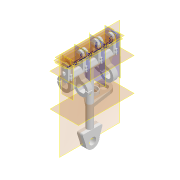
# Autodesk Inventor part: base_hand
Saved by Autodesk Inventor 2020.2 (Build 242310000, 310)
## iProperties
Created: 2020-04-08
Part Number: base_hand
Material: Generic
Document SubType Name: Modeling
Designer: Bardo91
Density: 1 g/cm^3
Appearance: Default
Author: Bardo91
Autodesk Inventor part; units mm, degrees
sketch "Sketch1" plane through (0, 0, 0) normal (1, 0, 0) x (0, 1, 0)
  line L0 (0, 0) -> (0, -22)
  line L1 (0, -22) -> (0, -44)
  line L2 (0, -44) -> (0, -66)
  line L3 (0, -22) -> (5, -22)
  line L4 (0, -44) -> (8, -44)
  line L5 (0, -66) -> (5, -66)
  dimension "d0" = 22
  dimension "d1" = 22
  dimension "d2" = 22
  dimension "d4" = 5
  dimension "d5" = 8
  dimension "d6" = 5
  constraints: 12 end point, 2 horizontal, 2 point on line, 1 perpendicular, 1 vertical
  measures "d0" distance of L0.start L0.end
  measures "d1" distance of L0.end L1.end
  measures "d2" distance of L1.end L2.end
  measures "d4" distance of L0.end L3.end
  measures "d5" distance of L1.end L4.end
  measures "d6" distance of L2.end L5.end
ref_plane "Work Plane1" through (0, 5, -22) normal (0, 0, 1) x (1, 0, 0)
ref_plane "Work Plane3" through (0, 5, -66) normal (0, 0, 1) x (1, 0, 0)
ref_plane "Work Plane2" through (0, 8, -44) normal (0, 0, 1) x (1, 0, 0)
ref_plane "Work Plane4" through (0, 0, 0) normal (0, 0, 1) x (1, 0, 0)
sketch "Sketch2" plane through (0, 0, 0) normal (0, 0, 1) x (1, 0, 0)
  circle A0 centre (0, 0) radius 1.5
  circle A1 centre (0, 0) radius 5
  line L0 (0, 0) -> (0, -15)
  circle A2 centre (0, -15) radius 5
  line L1 (5, -15) -> (5, 0)
  line L2 (-5, -15) -> (-5, 0)
  dimension "d7" = 3
  dimension "d8" = 10
  dimension "d80" = 15
  dimension "d81" = 10
  constraints: 6 end point, 4 point on circle, 3 centre point, 3 coincident, 2 tangent, 2 vertical, 1 parallel
  measures "d7" diameter of A0
  measures "d8" diameter of A1
  measures "d80" distance of L0.start L0.end
  measures "d81" diameter of A2
extrude "pinky_joint" add sketch "Sketch2" along normal mid plane 8
sketch "Sketch18" plane through (0, 0, 4) normal (0, 0, 1) x (1, 0, 0)
  line L0 (0, 0) -> (0, -6)
  line L1 (0, -6) -> (0, -9)
  line L2 (0, 0) -> (1.058, -6)
  line L3 (0, 0) -> (6.0926, 0) construction
  line L4 (1.058, -6) -> (0, -6)
  line L5 (1.058, -6) -> (1.5869, -9)
  line L6 (1.5869, -9) -> (0, -9)
  dimension "d82" = 6
  dimension "d83" = 3
  dimension "d84" = 80
  constraints: 14 end point, 2 horizontal, 2 point on line, 1 equal length, 1 parallel, 1 vertical
  measures "d82" distance of L0.start L0.end
  measures "d83" distance of L0.end L1.end
  measures "d84" angle of L2 L3
extrude "lock" add sketch "Sketch18" along normal blind 3 contours L4 L5 L6 L1
ref_plane "Work Plane5" through (0, 0, 0) normal (0, 0, 1) x (1, 0, 0)
mirror "Mirror1" about plane through (0, 0, 0) normal (0, 0, 1) of "lock"
chamfer "Chamfer1" distance 3 angle 45 2 edges at (0, -7.5, 4) (0, -7.5, -4)
ref_plane "Work Plane6" through (0, 5, 0) normal (0, 1, 0) x (-1, 0, 0)
sketch "Sketch19" plane through (0, 5, 0) normal (0, 1, 0) x (-1, 0, 0)
  line L0 (0, 0) -> (-3, 0)
  circle A0 centre (-3, 0) radius 1.25
  dimension "d90" = 3
  dimension "thread_hole" = 2.5
  constraints: 2 end point, 1 centre point, 1 coincident, 1 horizontal
  measures "d90" distance of L0.start L0.end
  measures "thread_hole" diameter of A0
extrude "thread_hole" cut sketch "Sketch19" against normal through all
sketch "Sketch20" plane through (0, 0, 0) normal (0, 1, 0) x (-1, 0, 0)
  line L0 (0, 0) -> (-3, 0)
  circle A0 centre (-3, 0) radius 1.25
  line L1 (-3, -1.25) -> (-5, -1.25)
  line L2 (-5, -4) -> (-5, 4) projected
  line L3 (-3, 1.25) -> (-5, 1.25)
  line L4 (0, 0) -> (0, 2.405)
  dimension "d94" = 3
  dimension "d95" = 2.5
  constraints: 8 end point, 2 horizontal, 2 point on circle, 2 point on line, 1 centre point, 1 coincident, 1 parallel, 1 vertical
  measures "d94" distance of L0.start L0.end
  measures "d95" diameter of A0
revolve "Revolution2" cut sketch "Sketch20" angle 180 about axis through (0, 0, 0) along (0, 0, 1)
sketch "Sketch22" plane through (5, -15, 4) normal (1, 0, 0) x (0, 0, -1)
  line L0 (8, 0) -> (0, 0) projected
  line L1 (4, 0) -> (4, 1)
  circle A0 centre (4, 1) radius 1
  line L2 (4, 1) -> (4, 5)
  circle A1 centre (4, 5) radius 1
  point P0 (4, 15)
  dimension "d100" = 1
  dimension "d101" = 2
  dimension "d104" = 4
  dimension "d105" = 2
  constraints: 4 end point, 2 centre point, 2 coincident, 2 vertical, 1 midpoint
  measures "d100" distance of L1.start L1.end
  measures "d101" diameter of A0
  measures "d104" distance of L2.start L2.end
  measures "d105" diameter of A1
extrude "pinky_flector_holder" cut sketch "Sketch22" against normal up to surface round surface about axis through (3, 5, 0) along (0, -1, 0) radius 1.25 far side no
sketch "Sketch23" plane through (0, 0, -4) normal (0, 0, -1) x (-1, 0, 0)
  arc A0 (-5, -15) -> (5, -15) centre (0, -15) ccw projected
  circle A1 centre (0, -15) radius 5
  point P0 (0, 0)
  constraints: 1 coincident, 3 other
extrude "finger_union" add sketch "Sketch23" along normal blind 66
sketch "Sketch24" plane through (-5, 0, -1.25) normal (0, 1, 0) x (1, 0, 0)
  arc A0 (2, -2.5) -> (2, 0) centre (2, -1.25) ccw projected
  circle A1 centre (2, -1.25) radius 1.25
  point P0 (5, -1.25)
  constraints: 1 coincident, 3 other
extrude "pinky_actuator_hole" cut sketch "Sketch24" against normal through all
ref_plane "Work Plane7" through (0, 5, -22) normal (0, 0, -1) x (-1, 0, 0)
sketch "Sketch25" plane through (0, 5, -22) normal (0, 0, -1) x (-1, 0, 0)
  arc A0 (5, -5) -> (-5, -5) centre (0, -5) ccw projected
  circle A1 centre (0, 0) radius 1.5
  circle A2 centre (0, 0) radius 5
  line L0 (5, -5) -> (5, -20) projected
  line L1 (5, 0) -> (5, -20)
  line L2 (-5, -20) -> (-5, -5) projected
  line L3 (-5, 0) -> (-5, -20)
  circle A3 centre (0, -20) radius 5 projected
  circle A4 centre (0, -20) radius 5
  point P0 (-5, -5)
  point P1 (5, -5)
  dimension "d112" = 3
  dimension "d113" = 10
  constraints: 4 end point, 3 point on circle, 2 centre point, 2 coincident, 2 collinear, 1 horizontal alignment, 2 other
  measures "d112" diameter of A1
  measures "d113" diameter of A2
extrude "ring_base" add sketch "Sketch25" along normal mid plane 8 contours L0 A3 L2 A0 A2 | A0 A2 L1 | A2 A0 A1 | A0 A1 A2 | A0 L3 A2
sketch "Sketch26" plane through (0, 5, -18) normal (0, 0, 1) x (1, 0, 0)
  line L0 (0, 0) -> (0, -6)
  line L1 (0, -6) -> (0, -9)
  line L2 (0, 0) -> (1.5869, -9)
  line L3 (0, 0) -> (9.1388, 0) construction
  line L4 (1.5869, -9) -> (0, -9)
  line L5 (0, -6) -> (1.058, -6)
  point P0 (0, -5)
  dimension "d116" = 6
  dimension "d117" = 3
  dimension "d118" = 80
  constraints: 12 end point, 2 horizontal, 2 vertical, 1 equal length, 1 parallel, 1 point on line
  measures "d116" distance of L0.start L0.end
  measures "d117" distance of L0.end L1.end
  measures "d118" angle of L2 L3
extrude "ring_lock" add sketch "Sketch26" along normal blind 3 contours L5 L2 L4 L1
mirror "Mirror2" about plane through (0, 5, -22) normal (0, 0, -1) of "ring_lock"
chamfer "Chamfer2" distance 3 angle 45 2 edges at (0, -2.5, -18) (0, -2.5, -26)
ref_plane "Work Plane8" through (0, 8, -44) normal (0, 0, -1) x (-1, 0, 0)
ref_plane "Work Plane9" through (0, 5, -66) normal (0, 0, -1) x (-1, 0, 0)
sketch "Sketch27" plane through (0, 8, -44) normal (0, 0, -1) x (-1, 0, 0)
  circle A0 centre (0, 0) radius 1.5
  circle A1 centre (0, 0) radius 5
  line L0 (5, -8) -> (5, -23) projected
  line L1 (5, 0) -> (5, -23)
  arc A2 (5, -23) -> (-5, -23) centre (0, -23) ccw projected
  line L2 (-5, 0) -> (-5, -23)
  point P0 (0, -8)
  point P1 (5, -8)
  dimension "d124" = 3
  dimension "d125" = 10
  constraints: 4 end point, 2 centre point, 2 point on circle, 2 vertical, 1 coincident, 1 tangent
  measures "d124" diameter of A0
  measures "d125" diameter of A1
extrude "middle_base" add sketch "Sketch27" along normal mid plane 8
ref_plane "Work Plane11" through (5, 8, -40) normal (0, 1, 0) x (-1, 0, 0)
ref_plane "Work Plane10" through (5, 5, -18) normal (0, 1, 0) x (-1, 0, 0)
sketch "Sketch28" plane through (0, 5, -66) normal (0, 0, -1) x (-1, 0, 0)
  circle A0 centre (0, 0) radius 1.5
  circle A1 centre (0, 0) radius 5
  line L0 (5, 3) -> (5, -20) projected
  line L1 (5, 0) -> (5, -20)
  line L2 (-5, -20) -> (-5, 3) projected
  line L3 (-5, 0) -> (-5, -20)
  arc A2 (5, -20) -> (-5, -20) centre (0, -20) ccw projected
  circle A3 centre (0, -20) radius 5
  point P0 (0, -5)
  dimension "d128" = 3
  dimension "d129" = 10
  constraints: 4 end point, 2 centre point, 2 coincident, 2 collinear, 2 point on circle, 2 point on line, 1 horizontal alignment, 1 tangent, 2 other
  measures "d128" diameter of A0
  measures "d129" diameter of A1
extrude "index_base" add sketch "Sketch28" along normal mid plane 8 contours A1 | L0 A2 L2 A1
sketch "Sketch39" plane through (5, 5, -18) normal (0, 1, 0) x (-1, 0, 0)
  line L0 (10, -8) -> (10, 0) projected
  line L1 (10, -4) -> (0, -4)
  line L2 (0, -8) -> (0, 0) projected
  line L3 (5, -4) -> (1.5, -4)
  circle A0 centre (1.5, -4) radius 1.25
  line L4 (1.5, -5.25) -> (0, -5.25)
  line L5 (1.5, -2.75) -> (0, -2.75)
  line L6 (5, -4) -> (5, -5.6429)
  line L7 (0, -5.25) -> (0, -2.75)
  point P0 (5, 18)
  dimension "d165" = 3.5
  dimension "d166" = 2.5
  constraints: 12 end point, 3 midpoint, 3 point on line, 2 perpendicular, 2 point on circle, 1 centre point, 1 coincident, 1 collinear, 1 tangent, 1 vertical
  measures "d165" distance of L3.start L3.end
  measures "d166" diameter of A0
revolve "ring_1" cut sketch "Sketch39" angle 180 about axis through (0, 5, -22) along (0, 0, 1)
sketch "Sketch40" plane through (3.5, 5, -20.75) normal (0, 1, 0) x (1, 0, 0)
  arc A0 (0, 2.5) -> (0, 0) centre (0, 1.25) ccw projected
  circle A1 centre (0, 1.25) radius 1.25
  point P0 (-3.5, -20.75)
  constraints: 1 coincident, 3 other
extrude "ring_2" cut sketch "Sketch40" against normal through all
sketch "Sketch41" plane through (5, -15, -26) normal (1, 0, 0) x (0, 0, -1)
  line L0 (0, 0) -> (-8, 0) projected
  line L1 (-4, 0) -> (-4, 1)
  line L2 (-4, 1) -> (-4, 5)
  circle A0 centre (-4, 5) radius 1
  circle A1 centre (-4, 1) radius 1
  point P0 (-26, 15)
  dimension "d170" = 1
  dimension "d171" = 4
  dimension "d172" = 2
  dimension "d173" = 2
  constraints: 4 end point, 2 centre point, 2 coincident, 1 midpoint, 1 point on line, 1 vertical
  measures "d170" distance of L1.start L1.end
  measures "d171" distance of L1.end L2.end
  measures "d172" diameter of A0
  measures "d173" diameter of A1
extrude "ring_3" cut sketch "Sketch41" against normal up to surface round surface about axis through (3.5, 5, -22) along (0, -1, 0) radius 1.25 far side no
sketch "Sketch42" plane through (-5, 5, -20.75) normal (0, 1, 0) x (1, 0, 0)
  arc A0 (1.5, 0) -> (1.5, 2.5) centre (1.5, 1.25) ccw projected
  circle A1 centre (1.5, 1.25) radius 1.25
  point P0 (5, -20.75)
  constraints: 1 coincident, 3 other
extrude "ring_4" cut sketch "Sketch42" against normal through all
sketch "Sketch30" plane through (5, 8, -40) normal (0, 1, 0) x (-1, 0, 0)
  line L0 (10, -8) -> (10, 0) projected
  line L1 (10, -4) -> (0, -4)
  line L2 (0, 0) -> (0, -8) projected
  line L3 (5, -4) -> (1.5, -4)
  circle A0 centre (1.5, -4) radius 1.25
  line L4 (1.5, -5.25) -> (0, -5.25)
  line L5 (1.5, -2.75) -> (0, -2.75)
  line L6 (5, -4) -> (5, -4.8662)
  point P0 (5, 40)
  dimension "d135" = 3.5
  dimension "d136" = 2.5
  constraints: 10 end point, 3 midpoint, 3 point on line, 2 point on circle, 1 centre point, 1 coincident, 1 parallel, 1 perpendicular, 1 tangent, 1 vertical
  measures "d135" distance of L3.start L3.end
  measures "d136" diameter of A0
revolve "middle_1" cut sketch "Sketch30" angle 180 about axis through (0, 8, -44) along (0, 0, 1)
sketch "Sketch34" plane through (3.5, 8, -45.25) normal (0, 1, 0) x (1, 0, 0)
  arc A0 (0, 0) -> (0, -2.5) centre (0, -1.25) ccw projected
  circle A1 centre (0, -1.25) radius 1.25
  point P0 (-3.5, -45.25)
  point P1 (0, -2.5)
  constraints: 1 coincident, 3 other
extrude "middle_2" cut sketch "Sketch34" against normal through all
sketch "Sketch35" plane through (5, -15, -48) normal (1, 0, 0) x (0, 0, -1)
  line L0 (0, 0) -> (-8, 0) projected
  line L1 (-4, 0) -> (-4, 1)
  line L2 (-4, 1) -> (-4, 5)
  circle A0 centre (-4, 1) radius 1
  circle A1 centre (-4, 5) radius 1
  point P0 (-48, 15)
  dimension "d151" = 1
  dimension "d152" = 4
  dimension "d153" = 2
  dimension "d154" = 2
  constraints: 4 end point, 2 centre point, 2 coincident, 1 midpoint, 1 point on line, 1 vertical
  measures "d151" distance of L1.start L1.end
  measures "d152" distance of L1.end L2.end
  measures "d153" diameter of A0
  measures "d154" diameter of A1
extrude "middle_3" cut sketch "Sketch35" against normal up to surface round surface about axis through (3.5, 8, -44) along (0, -1, 0) radius 1.25 far side no
sketch "Sketch43" plane through (-5, 8, -45.25) normal (0, 1, 0) x (1, 0, 0)
  arc A0 (1.5, -2.5) -> (1.5, 0) centre (1.5, -1.25) ccw projected
  circle A1 centre (1.5, -1.25) radius 1.25
  point P0 (5, -45.25)
  point P1 (1.5, 0)
  constraints: 1 centre point, 1 coincident
extrude "middle_4" cut sketch "Sketch43" against normal through all
sketch "Sketch31" plane through (5, 5, -18) normal (0, 1, 0) x (-1, 0, 0)
  line L0 (10, -44) -> (10, -52) projected
  line L1 (10, -48) -> (0, -48)
  line L2 (0, -52) -> (0, -44) projected
  line L3 (5, -48) -> (1.5, -48)
  circle A0 centre (1.5, -48) radius 1.25
  line L4 (1.5, -49.25) -> (0, -49.25)
  line L5 (1.5, -46.75) -> (0, -46.75)
  line L6 (5, -48) -> (5, -46.2742)
  point P0 (5, 18)
  dimension "d138" = 3.5
  dimension "d139" = 2.5
  constraints: 10 end point, 3 midpoint, 3 point on line, 2 perpendicular, 2 point on circle, 1 centre point, 1 coincident, 1 tangent, 1 vertical
  measures "d138" distance of L3.start L3.end
  measures "d139" diameter of A0
revolve "index_1" cut sketch "Sketch31" angle 180 about axis through (0, 5, -66) along (0, 0, 1)
sketch "Sketch36" plane through (3.5, 5, -64.75) normal (0, 1, 0) x (1, 0, 0)
  arc A0 (0, 2.5) -> (0, 0) centre (0, 1.25) ccw projected
  circle A1 centre (0, 1.25) radius 1.25
  point P0 (-3.5, -64.75)
  constraints: 1 coincident, 3 other
extrude "index_2" cut sketch "Sketch36" against normal through all
sketch "Sketch37" plane through (5, -15, -70) normal (1, 0, 0) x (0, 0, -1)
  line L0 (0, 0) -> (-8, 0) projected
  line L1 (-4, 0) -> (-4, 1)
  line L2 (-4, 1) -> (-4, 5)
  circle A0 centre (-4, 5) radius 1
  circle A1 centre (-4, 1) radius 1
  point P0 (-70, 15)
  dimension "d159" = 1
  dimension "d160" = 4
  dimension "d161" = 2
  dimension "d162" = 2
  constraints: 4 end point, 2 centre point, 2 coincident, 1 midpoint, 1 point on line, 1 vertical
  measures "d159" distance of L1.start L1.end
  measures "d160" distance of L1.end L2.end
  measures "d161" diameter of A0
  measures "d162" diameter of A1
extrude "index_3" cut sketch "Sketch37" against normal up to surface round surface about axis through (3.5, 5, -66) along (0, -1, 0) radius 1.25 far side no
sketch "Sketch44" plane through (-5, 5, -64.75) normal (0, 1, 0) x (1, 0, 0)
  arc A0 (1.5, 0) -> (1.5, 2.5) centre (1.5, 1.25) ccw projected
  circle A1 centre (1.5, 1.25) radius 1.25
  point P0 (5, -64.75)
  point P1 (1.5, 0)
  constraints: 1 coincident, 3 other
extrude "index_4" cut sketch "Sketch44" against normal through all
sketch "Sketch46" plane through (0, 5, -18) normal (0, 0, 1) x (1, 0, 0)
  arc A0 (-5, -20) -> (5, -20) centre (0, -20) ccw projected
  line L0 (0, -20) -> (0, -35)
  line L1 (0, -35) -> (9, -35)
  circle A1 centre (9, -35) radius 6
  circle A2 centre (9, -35) radius 10
  line L2 (9, -35) -> (9, -30)
  line L3 (9, -30) -> (12.3166, -30)
  line L4 (9, -30) -> (5.6834, -30)
  line L5 (9, -35) -> (9, -40)
  line L6 (9, -40) -> (12.3166, -40)
  line L7 (9, -40) -> (5.6834, -40)
  line L8 (9, -35) -> (9, -34.5)
  line L9 (9, -34.5) -> (18.9875, -34.5)
  line L10 (9, -35) -> (9, -35.5)
  line L11 (9, -35.5) -> (18.9875, -35.5)
  line L12 (9, -25) -> (5, -20)
  line L13 (-1, -35) -> (-5, -20)
  point P0 (0, -5)
  point P1 (14.9791, -34.5)
  point P2 (14.9791, -35.5)
  point P3 (-4.3361, -22.4896)
  dimension "d187" = 15
  dimension "d188" = 9
  dimension "d189" = 12
  dimension "d190" = 20
  dimension "d191" = 5
  dimension "d192" = 5
  dimension "d193" = 0.5
  dimension "d194" = 0.5
  constraints: 28 end point, 9 point on circle, 5 perpendicular, 5 point on line, 2 centre point, 2 coincident, 2 vertical
  measures "d187" distance of L0.start L0.end
  measures "d188" distance of L0.end L1.end
  measures "d189" diameter of A1
  measures "d190" diameter of A2
  measures "d191" distance of L2.start L2.end
  measures "d192" distance of L2.start L5.end
  measures "d193" distance of L2.start L8.end
  measures "d194" distance of L2.start L10.end
sketch "Sketch51" plane through (0, 8, -48) normal (0, 0, -1) x (-1, 0, 0)
  arc A0 (-4.9962, -22.8052) -> (-4.9944, -22.7631) centre (0, -23) ccw
  line L0 (0, -23) -> (0, -38)
  line L1 (0, -38) -> (-9, -38)
  circle A1 centre (-9, -38) radius 6
  circle A2 centre (-9, -38) radius 10
  line L2 (-9, -38) -> (-9, -33)
  line L3 (-9, -33) -> (-5.6834, -33)
  line L4 (-9, -33) -> (-12.3166, -33)
  line L5 (-9, -38) -> (-9, -43)
  line L6 (-9, -43) -> (-5.6834, -43)
  line L7 (-9, -43) -> (-12.3166, -43)
  line L8 (-9, -38) -> (-9, -37.5)
  line L9 (-9, -38) -> (-9, -38.5)
  arc A3 (-5, -23) -> (5, -23) centre (0, -23) ccw projected
  line L10 (-9, -28) -> (-5, -23)
  line L11 (1, -38) -> (5, -23)
  line L12 (-9, -38.5) -> (-18.9875, -38.5)
  line L13 (-9, -37.5) -> (-18.9875, -37.5)
  point P0 (0, -5)
  point P1 (0, -5)
  point P2 (0.9875, -37.5)
  point P3 (0.9875, -38.5)
  point P4 (-5, -23)
  point P5 (5, -23)
  point P6 (4.3361, -25.4896)
  point P7 (-14.9791, -37.5)
  point P8 (-14.9791, -38.5)
  dimension "d227" = 15
  dimension "d229" = 12
  dimension "d230" = 20
  dimension "d231" = 5
  dimension "d232" = 5
  dimension "d233" = 0.5
  dimension "d234" = 0.5
  dimension "d235" = 5
  dimension "d237" = 9
  constraints: 28 end point, 12 point on circle, 5 point on line, 4 coincident, 3 centre point, 3 perpendicular, 2 vertical, 1 horizontal
  measures "d227" distance of L0.start L0.end
  measures "d229" diameter of A1
  measures "d230" diameter of A2
  measures "d231" distance of L2.start L2.end
  measures "d232" distance of L2.start L5.end
  measures "d233" distance of L2.start L8.end
  measures "d234" distance of L2.start L9.end
  measures "d235" radius of A0
  measures "d237" distance of L0.end L1.end
extrude "pinky_motor" add sketch "Sketch46" along normal blind 7 contours A0 L0 A2 L13 | A0 L12 A2 L0 | A2 L0 L1 A1 L11 | A2 L9 A1 L1 L0 | A1 L7 L6 | A1 L3 L4
extrude "index_motor" add sketch "Sketch51" along normal blind 7 contours A0 L0 A2 L10 | A0 L11 A2 L0 | A2 L0 L1 A1 L13 | A2 L12 A1 L1 L0 | A1 L7 L6
sketch "Sketch52" plane through (0, 5, -62) normal (0, 0, 1) x (1, 0, 0)
  arc A0 (-4.9995, -20.0687) -> (4.9995, -20.0687) centre (0, -20) ccw
  line L0 (0, -20) -> (0, -35)
  line L1 (0, -35) -> (-9, -35)
  circle A1 centre (-9, -35) radius 6
  circle A2 centre (-9, -35) radius 10
  line L2 (-9, -35) -> (-9, -30)
  line L3 (-9, -30) -> (-5.6834, -30)
  line L4 (-9, -30) -> (-12.3166, -30)
  line L5 (-9, -35) -> (-9, -40)
  line L6 (-9, -40) -> (-5.6834, -40)
  line L7 (-9, -40) -> (-12.3166, -40)
  line L8 (-9, -35) -> (-9, -34.5)
  line L9 (-9, -35) -> (-9, -35.5)
  arc A3 (-4.3361, -22.4896) -> (5, -20) centre (0, -20) ccw projected
  line L10 (5, -20) -> (9, -25) projected
  line L11 (1, -35) -> (5, -20)
  line L12 (-1, -35) -> (-4.3361, -22.4896) projected
  line L13 (-4.3361, -22.4896) -> (-8.7782, -25.0025)
  line L14 (-9, -35.5) -> (-18.9875, -35.5)
  line L15 (-9, -34.5) -> (-18.9875, -34.5)
  point P0 (0, -5)
  point P1 (0, -5)
  point P2 (0.9875, -34.5)
  point P3 (0.9875, -35.5)
  point P4 (11.9791, -34.5)
  point P5 (11.9791, -35.5)
  point P6 (-4.9558, -20.6637)
  point P7 (4.3361, -22.4896)
  point P8 (-4.3361, -22.4896)
  point P9 (-3.1658, -26.8783)
  point P10 (-14.9791, -34.5)
  point P11 (-14.9791, -35.5)
  dimension "d246" = 15
  dimension "d248" = 12
  dimension "d249" = 20
  dimension "d250" = 5
  dimension "d251" = 5
  dimension "d252" = 0.5
  dimension "d253" = 0.5
  dimension "d254" = 5
  dimension "d256" = 9
  constraints: 28 end point, 13 point on circle, 6 point on line, 4 coincident, 3 centre point, 3 perpendicular, 2 vertical, 1 horizontal
  measures "d246" distance of L0.start L0.end
  measures "d248" diameter of A1
  measures "d249" diameter of A2
  measures "d250" distance of L2.start L2.end
  measures "d251" distance of L2.start L5.end
  measures "d252" distance of L2.start L8.end
  measures "d253" distance of L2.start L9.end
  measures "d254" radius of A0
  measures "d256" distance of L0.end L1.end
extrude "ring_motor" add sketch "Sketch52" along normal blind 7 contours A0 L0 A2 L12 | A0 L11 A2 L0 | L12 L1 A1 L15 A2 | A2 L0 L1 L12 | A2 L14 A1 L1 L0 | L3 L4 A1
sketch "Sketch53" plane through (0, 0, -4) normal (0, 0, -1) x (-1, 0, 0)
  arc A0 (-2, -15) -> (2, -15) centre (0, -15) ccw
  line L0 (0, -15) -> (0, -30)
  line L1 (0, -30) -> (9, -30)
  circle A1 centre (9, -30) radius 6
  circle A2 centre (9, -30) radius 10
  line L2 (9, -30) -> (9, -25)
  line L3 (9, -25) -> (12.3166, -25)
  line L4 (9, -25) -> (5.6834, -25)
  line L5 (9, -30) -> (9, -35)
  line L6 (9, -35) -> (12.3166, -35)
  line L7 (9, -35) -> (5.6834, -35)
  line L8 (9, -30) -> (9, -29.5)
  line L9 (9, -29.5) -> (18.9875, -29.5)
  line L10 (9, -30) -> (9, -30.5)
  line L11 (9, -30.5) -> (18.9875, -30.5)
  line L12 (9, -20) -> (2, -15)
  line L13 (-1, -30) -> (-2, -15)
  arc A3 (-5, -15) -> (5, -15) centre (0, -15) ccw projected
  point P0 (0, 0)
  point P1 (11.9791, -34.5)
  point P2 (11.9791, -35.5)
  point P3 (-4.9558, -20.6637)
  point P4 (-0.0209, -34.5)
  point P5 (4.9558, -20.6637)
  point P6 (-4.9558, -20.6637)
  point P7 (-4.6607, -25.0901)
  point P8 (-0.0209, -35.5)
  point P9 (0, -5)
  point P10 (11.9791, -34.5)
  point P11 (11.9791, -35.5)
  point P12 (-4.9558, -20.6637)
  point P13 (14.9791, -29.5)
  point P14 (-1.9823, -15.2655)
  point P15 (14.9791, -30.5)
  dimension "d270" = 15
  dimension "d271" = 9
  dimension "d272" = 12
  dimension "d273" = 20
  dimension "d274" = 5
  dimension "d275" = 5
  dimension "d276" = 0.5
  dimension "d277" = 0.5
  constraints: 28 end point, 11 point on circle, 5 perpendicular, 5 point on line, 4 coincident, 3 centre point, 2 vertical
  measures "d270" distance of L0.start L0.end
  measures "d271" distance of L0.end L1.end
  measures "d272" diameter of A1
  measures "d273" diameter of A2
  measures "d274" distance of L2.start L2.end
  measures "d275" distance of L2.start L5.end
  measures "d276" distance of L2.start L8.end
  measures "d277" distance of L2.start L10.end
extrude "middle_motor" add sketch "Sketch53" along normal blind 7 contours A0 L0 A3 L13 | A0 L12 A3 L0 | A3 L0 A2 L13 | A3 L12 A2 L0 | A2 L0 L1 A1 L11 | A2 L9 A1 L1 L0 | A1 L7 L6 | A1 L3 L4
sketch "Sketch54" plane through (0, 8, -40) normal (0, 0, 1) x (1, 0, 0)
  line L0 (0, 0) -> (0, -6)
  line L1 (0, -6) -> (0, -9)
  circle A0 centre (0, 0) radius 1.5 projected
  line L2 (0, 0) -> (1.5869, -9)
  line L3 (0, 0) -> (9.1388, 0) construction
  line L4 (1.5869, -9) -> (0, -9)
  line L5 (-2.25, -3) -> (-2.25, -27.4651) projected
  line L6 (0, -6) -> (1.058, -6)
  point P0 (0, -8)
  dimension "d282" = 6
  dimension "d283" = 3
  dimension "d284" = 80
  constraints: 12 end point, 2 point on line, 1 equal length, 1 horizontal, 1 parallel, 1 perpendicular, 1 vertical
  measures "d282" distance of L0.start L0.end
  measures "d283" distance of L0.end L1.end
  measures "d284" angle of L2 L3
extrude "lock_middle" add sketch "Sketch54" along normal blind 3 contours L6 L2 L4 L1
mirror "Mirror3" about plane through (0, 8, -44) normal (0, 0, -1) of "lock_middle"
chamfer "Chamfer3" distance 3 angle 45 2 edges at (0, 0.5, -40) (0, 0.5, -48)
sketch "Sketch55" plane through (0, 5, -62) normal (0, 0, 1) x (1, 0, 0)
  line L0 (0, 0) -> (0, -6)
  line L1 (0, 0) -> (6, 0) construction
  line L2 (0, -6) -> (0, -9)
  line L3 (0, 0) -> (1.5869, -9)
  line L4 (0, 0) -> (9.1388, 0) construction
  line L5 (1.5869, -9) -> (0, -9)
  line L6 (-2.25, 0) -> (-2.25, -24.4651) projected
  line L7 (0, -6) -> (1.058, -6)
  point P0 (0, -5)
  dimension "d290" = 6
  dimension "d291" = 90
  dimension "d292" = 3
  dimension "d293" = 80
  constraints: 14 end point, 2 equal length, 2 horizontal, 2 point on line, 1 parallel, 1 perpendicular, 1 vertical
  measures "d290" distance of L0.start L0.end
  measures "d291" angle of L0 L1
  measures "d292" distance of L0.end L2.end
  measures "d293" angle of L3 L4
extrude "lock_index" add sketch "Sketch55" along normal blind 3 contours L7 L3 L5 L2
mirror "Mirror4" about plane through (0, 5, -66) normal (0, 0, -1) of "lock_index"
chamfer "Chamfer4" distance 3 angle 45 2 edges at (0, -2.5, -70) (0, -2.5, -62)
sketch "Sketch56" plane through (5, -15, 4) normal (1, 0, 0) x (0, 0, -1)
  circle A0 centre (4, 5) radius 1 projected
  circle A1 centre (4, 5) radius 1
  circle A2 centre (4, 5) radius 2
  circle A3 centre (4, 1) radius 1 projected
  circle A4 centre (4, 1) radius 1
  circle A5 centre (4, 1) radius 2
  circle A6 centre (26, 5) radius 1 projected
  circle A7 centre (26, 5) radius 1
  circle A8 centre (26, 5) radius 2
  circle A9 centre (26, 1) radius 1 projected
  circle A10 centre (26, 1) radius 1
  circle A11 centre (26, 1) radius 2
  circle A12 centre (48, 5) radius 1 projected
  circle A13 centre (48, 5) radius 1
  circle A14 centre (48, 5) radius 2
  circle A15 centre (48, 1) radius 1 projected
  circle A16 centre (48, 1) radius 1
  circle A17 centre (48, 1) radius 2
  circle A18 centre (70, 5) radius 1 projected
  circle A19 centre (70, 5) radius 1
  circle A20 centre (70, 5) radius 2
  circle A21 centre (70, 1) radius 1 projected
  circle A22 centre (70, 1) radius 1
  circle A23 centre (70, 1) radius 2
  point P0 (4, 15)
  point P1 (4, 0)
  point P2 (26, 0)
  point P3 (48, 0)
  point P4 (70, 0)
  dimension "d299" = 4
  dimension "d300" = 4
  dimension "d301" = 4
  dimension "d302" = 4
  dimension "d303" = 4
  dimension "d304" = 4
  dimension "d305" = 4
  dimension "d306" = 4
  constraints: 16 centre point, 16 coincident, 4 vertical alignment
  measures "d299" diameter of A2
  measures "d300" diameter of A5
  measures "d301" diameter of A8
  measures "d302" diameter of A11
  measures "d303" diameter of A14
  measures "d304" diameter of A17
  measures "d305" diameter of A20
  measures "d306" diameter of A23
extrude "reinforcement_thread_screw" add sketch "Sketch56" along normal blind 2
ref_plane "Work Plane12" through (-5, -15, -70) normal (0, 1, 0) x (-1, 0, 0)
sketch "Sketch57" plane through (-5, -15, -70) normal (0, 1, 0) x (-1, 0, 0)
  line L0 (-10, 0) -> (-10, 74) projected
  line L1 (-10, 37) -> (0, 37)
  line L2 (0, 0) -> (0, 74) projected
  line L3 (0, 37) -> (-4.5, 37)
  circle A0 centre (-4.5, 37) radius 4.5
  point P0 (-5, 70)
  dimension "d309" = 4.5
  constraints: 4 end point, 2 midpoint, 1 centre point, 1 coincident, 1 point on line, 1 tangent
  measures "d309" distance of L1.end L3.end
extrude "spine_hand" add sketch "Sketch57" against normal blind 90
ref_plane "Work Plane13" through (-5, -63, -70) normal (0, 1, 0) x (-1, 0, 0)
sketch "Sketch58" plane through (-5, -63, -70) normal (0, 1, 0) x (-1, 0, 0)
  circle A0 centre (-4.5, 37) radius 4.5 projected
  line L0 (-4.5, 37) -> (-4.5, 7)
  line L1 (-10, 0) -> (0, 0) projected
  line L2 (-4.5, 7) -> (5.5, 7)
  circle A1 centre (5.5, 7) radius 6
  circle A2 centre (5.5, 7) radius 10
  line L3 (5.5, 7) -> (5.5, 12)
  line L4 (5.5, 12) -> (2.1834, 12)
  line L5 (5.5, 12) -> (8.8166, 12)
  line L6 (5.5, 7) -> (5.5, 2)
  line L7 (5.5, 2) -> (2.1834, 2)
  line L8 (5.5, 2) -> (8.8166, 2)
  line L9 (5.5, 7) -> (5.5, 6.5)
  line L10 (5.5, 6.5) -> (15.4875, 6.5)
  line L11 (5.5, 7) -> (5.5, 7.5)
  line L12 (5.5, 7.5) -> (15.4875, 7.5)
  line L13 (5.5, 7) -> (5.5, 22)
  circle A3 centre (5.5, 22) radius 6
  circle A4 centre (5.5, 22) radius 10
  line L14 (5.5, 22) -> (5.5, 17)
  line L15 (5.5, 17) -> (2.1834, 17)
  line L16 (5.5, 17) -> (8.8166, 17)
  line L17 (5.5, 22) -> (5.5, 27)
  line L18 (5.5, 27) -> (2.1834, 27)
  line L19 (5.5, 27) -> (8.8166, 27)
  line L20 (5.5, 22) -> (5.5, 22.5)
  line L21 (5.5, 22.5) -> (15.4875, 22.5)
  line L22 (5.5, 22) -> (5.5, 21.5)
  line L23 (5.5, 21.5) -> (15.4875, 21.5)
  line L24 (-1.7272, 40.5444) -> (11.7315, 29.821)
  line L25 (-8.9515, 36.3412) -> (-4.3922, 5.5359)
  point P0 (-5, 70)
  point P1 (11.4791, 7.5)
  point P2 (11.4791, 6.5)
  point P3 (-0.5435, 39.1438)
  point P4 (14.2922, 11.7641)
  point P5 (11.4791, 22.5)
  point P6 (-1.1144, 14.5)
  point P7 (5.5, 17)
  point P8 (5.5, 17)
  point P9 (12.1144, 14.5)
  point P10 (11.4791, 21.5)
  point P11 (-1.6958, 40.5195)
  dimension "d313" = 30
  dimension "d314" = 10
  dimension "d315" = 12
  dimension "d316" = 5
  dimension "d317" = 5
  dimension "d318" = 0.5
  dimension "d319" = 0.5
  dimension "d325" = 15
  dimension "d326" = 12
  dimension "d327" = 5
  dimension "d328" = 5
  dimension "d329" = 0.5
  dimension "d330" = 0.5
  constraints: 50 end point, 18 point on circle, 11 point on line, 10 perpendicular, 5 tangent, 4 centre point, 4 coincident, 2 vertical
  measures "d313" distance of L0.start L0.end
  measures "d314" distance of L0.end L2.end
  measures "d315" diameter of A1
  measures "d316" distance of L3.start L3.end
  measures "d317" distance of L3.start L6.end
  measures "d318" distance of L3.start L9.end
  measures "d319" distance of L3.start L11.end
  measures "d325" distance of L3.start L13.end
  measures "d326" diameter of A3
  measures "d327" distance of L14.start L14.end
  measures "d328" distance of L14.start L17.end
  measures "d329" distance of L14.start L20.end
  measures "d330" distance of L14.start L22.end
extrude "thumb_motor_" add sketch "Sketch58" against normal blind 5 contours A0 L24 A4 L0 | L0 A2 L25 A0 | A4 L21 A3 A2 | A4 A2 L0 | A2 L2 A1 L10 | A2 A4 A1 L2 | A2 A3 L13 A1 A4 | A3 L15 A2 | A2 L13 A3 | A4 L4 A1 | A1 L13 A4 | A4 A2 A3 L23 | L19 L18 A3 | L7 L8 A1 | L16 A3 A2 | A2 A3 L13 | A3 A2 A4 A1 L13 | A1 A4 L13 | A4 A1 L5 | A2 L12 A1 A4
sketch "Sketch59" plane through (-5, -63, -70) normal (0, 1, 0) x (1, 0, 0)
  arc A0 (-8.8166, -17) -> (-11.4791, -21.5) centre (-5.5, -22) ccw projected
  circle A1 centre (-5.5, -22) radius 6
  arc A2 (-2.1834, -27) -> (-2.1834, -17) centre (-5.5, -22) ccw projected
  circle A3 centre (-5.5, -22) radius 7
  line L0 (-11.4791, -22.5) -> (-15.4875, -22.5) projected
  line L1 (-12.4821, -22.5) -> (-11.5, -22.5)
  line L2 (-15.4875, -21.5) -> (-11.4791, -21.5) projected
  line L3 (-12.4821, -21.5) -> (-11.4791, -21.5)
  point P0 (5, -70)
  dimension "d331" = 14
  constraints: 4 end point, 3 point on circle, 3 point on line, 2 centre point, 2 coincident, 1 collinear
  measures "d331" diameter of A3
extrude "Extrusion41" add sketch "Sketch59" along normal blind 4 contours A0 L2 A3 L0 A1
ref_plane "Work Plane14" through (-0.5, -105, -33) normal (1, 0, 0) x (0, 1, 0)
sketch "Sketch61" plane through (-0.5, -105, -33) normal (1, 0, 0) x (0, 1, 0)
  line L0 (0, 4.5) -> (0, -4.5) projected
  line L1 (0, 0) -> (-5, 0)
  line L2 (-5, 0) -> (-15, 0)
  circle A0 centre (-5, 0) radius 5
  circle A1 centre (-5, 0) radius 10
  line L3 (5, 0) -> (10, 0)
  line L4 (10, 0) -> (10, 12.2251)
  line L5 (10, 15) -> (10, -12.2251)
  line L6 (7.3675, -14.1225) -> (-5, -10)
  line L7 (7.3675, 14.1225) -> (-5, 10)
  arc A2 (10, 12.2251) -> (7.3675, 14.1225) centre (8, 12.2251) ccw
  arc A3 (7.3675, -14.1225) -> (10, -12.2251) centre (8, -12.2251) ccw
  point P0 (105, 33)
  point P1 (10, -15)
  dimension "d341" = 5
  dimension "d342" = 10
  dimension "d343" = 5
  dimension "d344" = 15
  dimension "d345" = 30
  dimension "d348" = 2
  constraints: 14 end point, 8 point on circle, 8 point on line, 4 tangent, 3 centre point, 2 coincident, 1 equal radius, 1 horizontal, 1 horizontal alignment, 1 midpoint, 1 perpendicular, 2 other
  measures "d341" distance of L1.start L1.end
  measures "d342" distance of L1.end L2.end
  measures "d343" distance of L3.start L3.end
  measures "d344" distance of L3.end L5.start
  measures "d345" distance of L5.start point (10, -15)
  measures "d348" radius of A2
extrude "Extrusion42" add sketch "Sketch61" along normal mid plane 9
equation "\"d95\" = thread_hole"
body "Solid1"
